Autodesk Inventor part; units mm, degrees
(part 2 of 4)
sketch "Sketch11" plane through (0, 0, -1) normal (0, 0, -1) x (-1, 0, 0)
  line L0 (5.295, -1.6238) -> (2.667, -1.6238) construction
  line L1 (2.667, -1.6238) -> (2.667, -0.5776) construction
  line L2 (2.667, -0.5776) -> (5.295, -0.5776) construction
  line L3 (5.295, -0.5776) -> (5.295, -1.6238) construction
  spline S0 degree 2 poles (4.8882, -1.2818) (4.8882, -1.2425) (4.915, -1.176) (4.9413, -1.1521) knots 0 0 0 1 2 2 2
  spline S1 degree 2 poles (4.9413, -1.1521) (4.9676, -1.1282) (5.0398, -1.1019) (5.0924, -1.1019) knots 0 0 0 1 2 2 2
  spline S2 degree 2 poles (5.0924, -1.1019) (5.1484, -1.1023) (5.2286, -1.1205) (5.2549, -1.1323) knots 0 0 0 1 2 2 2
  line L4 (5.2549, -1.1323) -> (5.2549, -1.2413)
  line L5 (5.2549, -1.2413) -> (5.2436, -1.2413)
  spline S3 degree 2 poles (5.2436, -1.2413) (5.2338, -1.236) (5.2103, -1.2222) (5.1913, -1.2149) knots 0 0 0 1 2 2 2
  spline S4 degree 2 poles (5.1913, -1.2149) (5.1735, -1.208) (5.1366, -1.1987) (5.1143, -1.1987) knots 0 0 0 1 2 2 2
  spline S5 degree 2 poles (5.1143, -1.1987) (5.0949, -1.1987) (5.0495, -1.2084) (5.0357, -1.2214) knots 0 0 0 1 2 2 2
  spline S6 degree 2 poles (5.0357, -1.2214) (5.0256, -1.2315) (5.0142, -1.2563) (5.0142, -1.2769) knots 0 0 0 1 2 2 2
  spline S7 degree 2 poles (5.0142, -1.2769) (5.0142, -1.2948) (5.0288, -1.3199) (5.0406, -1.3276) knots 0 0 0 1 2 2 2
  spline S8 degree 2 poles (5.0406, -1.3276) (5.0576, -1.3389) (5.1062, -1.3454) (5.1236, -1.3454) knots 0 0 0 1 2 2 2
  spline S9 degree 2 poles (5.1236, -1.3454) (5.1512, -1.3454) (5.2035, -1.3365) (5.2225, -1.3316) knots 0 0 0 1 2 2 2
  line L6 (5.2225, -1.3316) -> (5.2334, -1.3316)
  line L7 (5.2334, -1.3316) -> (5.2334, -1.6124)
  line L8 (5.2334, -1.6124) -> (4.902, -1.6124)
  line L9 (4.902, -1.6124) -> (4.902, -1.518)
  line L10 (4.902, -1.518) -> (5.1147, -1.518)
  line L11 (5.1147, -1.518) -> (5.1147, -1.4349)
  spline S10 degree 2 poles (5.1147, -1.4349) (5.1046, -1.4358) (5.0766, -1.4366) (5.0689, -1.4366) knots 0 0 0 1 2 2 2
  spline S11 degree 2 poles (5.0689, -1.4366) (5.0329, -1.4366) (4.9721, -1.422) (4.9482, -1.407) knots 0 0 0 1 2 2 2
  spline S12 degree 2 poles (4.9482, -1.407) (4.9198, -1.3883) (4.8882, -1.3264) (4.8882, -1.2818) knots 0 0 0 1 2 2 2
  spline S13 degree 2 poles (4.4401, -1.2514) (4.4401, -1.2194) (4.4668, -1.1639) (4.4924, -1.1436) knots 0 0 0 1 2 2 2
  spline S14 degree 2 poles (4.4924, -1.1436) (4.5179, -1.1234) (4.5912, -1.1007) (4.6386, -1.1007) knots 0 0 0 1 2 2 2
  spline S15 degree 2 poles (4.6386, -1.1007) (4.6893, -1.1007) (4.765, -1.1238) (4.7894, -1.1436) knots 0 0 0 1 2 2 2
  spline S16 degree 2 poles (4.7894, -1.1436) (4.8133, -1.1635) (4.836, -1.2174) (4.836, -1.2473) knots 0 0 0 1 2 2 2
  spline S17 degree 2 poles (4.836, -1.2473) (4.836, -1.2903) (4.7885, -1.3474) (4.7436, -1.3665) knots 0 0 0 1 2 2 2
  line L12 (4.7436, -1.3665) -> (4.7436, -1.3685)
  spline S18 degree 2 poles (4.7436, -1.3685) (4.7877, -1.39) (4.8226, -1.4512) (4.8226, -1.4888) knots 0 0 0 1 2 2 2
  spline S19 degree 2 poles (4.8226, -1.4888) (4.8226, -1.5164) (4.7983, -1.5646) (4.7744, -1.5836) knots 0 0 0 1 2 2 2
  spline S20 degree 2 poles (4.7744, -1.5836) (4.7513, -1.6019) (4.6812, -1.6238) (4.6374, -1.6238) knots 0 0 0 1 2 2 2
  spline S21 degree 2 poles (4.6374, -1.6238) (4.5912, -1.6238) (4.5223, -1.6039) (4.5001, -1.5877) knots 0 0 0 1 2 2 2
  spline S22 degree 2 poles (4.5001, -1.5877) (4.4774, -1.5715) (4.4531, -1.5245) (4.4531, -1.4973) knots 0 0 0 1 2 2 2
  spline S23 degree 2 poles (4.4531, -1.4973) (4.4531, -1.4617) (4.4944, -1.4046) (4.5369, -1.3847) knots 0 0 0 1 2 2 2
  line L13 (4.5369, -1.3847) -> (4.5369, -1.3831)
  spline S24 degree 2 poles (4.5369, -1.3831) (4.4871, -1.3628) (4.4401, -1.2972) (4.4401, -1.2514) knots 0 0 0 1 2 2 2
  spline S25 degree 2 poles (4.5641, -1.2461) (4.5641, -1.2708) (4.5851, -1.2968) (4.6192, -1.3134) knots 0 0 0 1 2 2 2
  spline S26 degree 2 poles (4.6192, -1.3134) (4.6289, -1.3178) (4.6658, -1.332) (4.68, -1.3381) knots 0 0 0 1 2 2 2
  spline S27 degree 2 poles (4.68, -1.3381) (4.6929, -1.3251) (4.7136, -1.2862) (4.7136, -1.2631) knots 0 0 0 1 2 2 2
  spline S28 degree 2 poles (4.7136, -1.2631) (4.7136, -1.2283) (4.669, -1.1866) (4.633, -1.1866) knots 0 0 0 1 2 2 2
  spline S29 degree 2 poles (4.633, -1.1866) (4.6228, -1.1866) (4.5977, -1.193) (4.588, -1.1995) knots 0 0 0 1 2 2 2
  spline S30 degree 2 poles (4.588, -1.1995) (4.577, -1.2072) (4.5641, -1.2283) (4.5641, -1.2461) knots 0 0 0 1 2 2 2
  spline S31 degree 2 poles (4.575, -1.4828) (4.575, -1.5083) (4.6086, -1.5387) (4.6374, -1.5387) knots 0 0 0 1 2 2 2
  spline S32 degree 2 poles (4.6374, -1.5387) (4.665, -1.5387) (4.6986, -1.5111) (4.6986, -1.4909) knots 0 0 0 1 2 2 2
  spline S33 degree 2 poles (4.6986, -1.4909) (4.6986, -1.471) (4.6783, -1.4463) (4.6569, -1.4362) knots 0 0 0 1 2 2 2
  spline S34 degree 2 poles (4.6569, -1.4362) (4.6475, -1.4313) (4.6216, -1.4212) (4.6001, -1.4131) knots 0 0 0 1 2 2 2
  spline S35 degree 2 poles (4.6001, -1.4131) (4.5872, -1.4301) (4.575, -1.4621) (4.575, -1.4828) knots 0 0 0 1 2 2 2
  line L14 (3.9948, -1.2291) -> (4.0625, -1.2291)
  line L15 (4.0625, -1.2291) -> (4.0625, -1.1112)
  line L16 (4.0625, -1.1112) -> (4.1836, -1.1112)
  line L17 (4.1836, -1.1112) -> (4.1836, -1.2291)
  line L18 (4.1836, -1.2291) -> (4.404, -1.2291)
  line L19 (4.404, -1.2291) -> (4.404, -1.3223)
  line L20 (4.404, -1.3223) -> (4.1877, -1.6124)
  line L21 (4.1877, -1.6124) -> (4.0625, -1.6124)
  line L22 (4.0625, -1.6124) -> (4.0625, -1.3191)
  line L23 (4.0625, -1.3191) -> (3.9948, -1.3191)
  line L24 (3.9948, -1.3191) -> (3.9948, -1.2291)
  line L25 (4.1836, -1.3191) -> (4.1836, -1.4892)
  line L26 (4.1836, -1.4892) -> (4.3104, -1.3191)
  line L27 (4.3104, -1.3191) -> (4.1836, -1.3191)
  point P0 (0, 0)
  constraints: 2 other
extrude "Extrusion11" add sketch "Sketch11" along normal blind 0.02 bodies 8
sketch "Sketch12" plane through (0, 0, 0) normal (0, 0, -1) x (-1, 0, 0)
  line L0 (3.7, 4.96) -> (5.6, 4.96)
  line L1 (5.6, 4.96) -> (5.6, 5.76)
  line L2 (5.6, 5.76) -> (3.7, 5.76)
  line L3 (3.7, 5.76) -> (3.7, 4.96)
  line L4 (3.6421, 4.9021) -> (3.6421, 5.8179)
  line L5 (5.6579, 5.8179) -> (5.6579, 4.9021)
  line L6 (5.7362, 4.8238) -> (5.7362, 5.8962)
  line L7 (3.5638, 5.8962) -> (3.5638, 4.8238)
  line L8 (4.75, 4.8238) -> (4.75, 4.9021)
  line L9 (4.55, 4.8238) -> (4.55, 4.9021)
  line L10 (4.75, 5.8179) -> (4.75, 5.8962)
  line L11 (4.55, 5.8179) -> (4.55, 5.8962)
  line L12 (3.6421, 5.8179) -> (4.55, 5.8179)
  line L13 (4.75, 5.8179) -> (5.6579, 5.8179)
  line L14 (5.7362, 5.8962) -> (4.75, 5.8962)
  line L15 (4.55, 5.8962) -> (3.5638, 5.8962)
  line L16 (5.6579, 4.9021) -> (4.75, 4.9021)
  line L17 (4.55, 4.9021) -> (3.6421, 4.9021)
  line L18 (3.5638, 4.8238) -> (4.55, 4.8238)
  line L19 (4.75, 4.8238) -> (5.7362, 4.8238)
  line L20 (3.6421, 3.5421) -> (3.6421, 4.4579)
  line L21 (5.6579, 4.4579) -> (5.6579, 3.5421)
  line L22 (5.7362, 3.4638) -> (5.7362, 4.5362)
  line L23 (3.5638, 4.5362) -> (3.5638, 3.4638)
  line L24 (4.75, 3.4638) -> (4.75, 3.5421)
  line L25 (4.55, 3.4638) -> (4.55, 3.5421)
  line L26 (4.75, 4.4579) -> (4.75, 4.5362)
  line L27 (4.55, 4.4579) -> (4.55, 4.5362)
  line L28 (3.6421, 4.4579) -> (4.55, 4.4579)
  line L29 (4.75, 4.4579) -> (5.6579, 4.4579)
  line L30 (5.7362, 4.5362) -> (4.75, 4.5362)
  line L31 (4.55, 4.5362) -> (3.5638, 4.5362)
  line L32 (5.6579, 3.5421) -> (4.75, 3.5421)
  line L33 (4.55, 3.5421) -> (3.6421, 3.5421)
  line L34 (3.5638, 3.4638) -> (4.55, 3.4638)
  line L35 (4.75, 3.4638) -> (5.7362, 3.4638)
  line L36 (3.6421, 2.2021) -> (3.6421, 3.1179)
  line L37 (5.6579, 3.1179) -> (5.6579, 2.2021)
  line L38 (5.7362, 2.1238) -> (5.7362, 3.1962)
  line L39 (3.5638, 3.1962) -> (3.5638, 2.1238)
  line L40 (4.75, 2.1238) -> (4.75, 2.2021)
  line L41 (4.55, 2.1238) -> (4.55, 2.2021)
  line L42 (4.75, 3.1179) -> (4.75, 3.1962)
  line L43 (4.55, 3.1179) -> (4.55, 3.1962)
  line L44 (3.6421, 3.1179) -> (4.55, 3.1179)
  line L45 (4.75, 3.1179) -> (5.6579, 3.1179)
  line L46 (5.7362, 3.1962) -> (4.75, 3.1962)
  line L47 (4.55, 3.1962) -> (3.5638, 3.1962)
  line L48 (5.6579, 2.2021) -> (4.75, 2.2021)
  line L49 (4.55, 2.2021) -> (3.6421, 2.2021)
  line L50 (3.5638, 2.1238) -> (4.55, 2.1238)
  line L51 (4.75, 2.1238) -> (5.7362, 2.1238)
  line L52 (3.6421, 0.8621) -> (3.6421, 1.7779)
  line L53 (5.6579, 1.7779) -> (5.6579, 0.8621)
  line L54 (5.7362, 0.7838) -> (5.7362, 1.8562)
  line L55 (3.5638, 1.8562) -> (3.5638, 0.7838)
  line L56 (4.75, 0.7838) -> (4.75, 0.8621)
  line L57 (4.55, 0.7838) -> (4.55, 0.8621)
  line L58 (4.75, 1.7779) -> (4.75, 1.8562)
  line L59 (4.55, 1.7779) -> (4.55, 1.8562)
  line L60 (3.6421, 1.7779) -> (4.55, 1.7779)
  line L61 (4.75, 1.7779) -> (5.6579, 1.7779)
  line L62 (5.7362, 1.8562) -> (4.75, 1.8562)
  line L63 (4.55, 1.8562) -> (3.5638, 1.8562)
  line L64 (5.6579, 0.8621) -> (4.75, 0.8621)
  line L65 (4.55, 0.8621) -> (3.6421, 0.8621)
  line L66 (3.5638, 0.7838) -> (4.55, 0.7838)
  line L67 (4.75, 0.7838) -> (5.7362, 0.7838)
  line L68 (3.6421, -0.4779) -> (3.6421, 0.4379)
  line L69 (5.6579, 0.4379) -> (5.6579, -0.4779)
  line L70 (5.7362, -0.5562) -> (5.7362, 0.5162)
  line L71 (3.5638, 0.5162) -> (3.5638, -0.5562)
  line L72 (4.75, -0.5562) -> (4.75, -0.4779)
  line L73 (4.55, -0.5562) -> (4.55, -0.4779)
  line L74 (4.75, 0.4379) -> (4.75, 0.5162)
  line L75 (4.55, 0.4379) -> (4.55, 0.5162)
  line L76 (3.6421, 0.4379) -> (4.55, 0.4379)
  line L77 (4.75, 0.4379) -> (5.6579, 0.4379)
  line L78 (5.7362, 0.5162) -> (4.75, 0.5162)
  line L79 (4.55, 0.5162) -> (3.5638, 0.5162)
  line L80 (5.6579, -0.4779) -> (4.75, -0.4779)
  line L81 (4.55, -0.4779) -> (3.6421, -0.4779)
  line L82 (3.5638, -0.5562) -> (4.55, -0.5562)
  line L83 (4.75, -0.5562) -> (5.7362, -0.5562)
  line L84 (3.6421, -1.8179) -> (3.6421, -0.9021)
  line L85 (5.6579, -0.9021) -> (5.6579, -1.8179)
  line L86 (5.7362, -1.8962) -> (5.7362, -0.8238)
  line L87 (3.5638, -0.8238) -> (3.5638, -1.8962)
  line L88 (4.75, -1.8962) -> (4.75, -1.8179)
  line L89 (4.55, -1.8962) -> (4.55, -1.8179)
  line L90 (4.75, -0.9021) -> (4.75, -0.8238)
  line L91 (4.55, -0.9021) -> (4.55, -0.8238)
  line L92 (3.6421, -0.9021) -> (4.55, -0.9021)
  line L93 (4.75, -0.9021) -> (5.6579, -0.9021)
  line L94 (5.7362, -0.8238) -> (4.75, -0.8238)
  line L95 (4.55, -0.8238) -> (3.5638, -0.8238)
  line L96 (5.6579, -1.8179) -> (4.75, -1.8179)
  line L97 (4.55, -1.8179) -> (3.6421, -1.8179)
  line L98 (3.5638, -1.8962) -> (4.55, -1.8962)
  line L99 (4.75, -1.8962) -> (5.7362, -1.8962)
  line L100 (3.6421, -3.1579) -> (3.6421, -2.2421)
  line L101 (5.6579, -2.2421) -> (5.6579, -3.1579)
  line L102 (5.7362, -3.2362) -> (5.7362, -2.1638)
  line L103 (3.5638, -2.1638) -> (3.5638, -3.2362)
  line L104 (4.75, -3.2362) -> (4.75, -3.1579)
  line L105 (4.55, -3.2362) -> (4.55, -3.1579)
  line L106 (4.75, -2.2421) -> (4.75, -2.1638)
  line L107 (4.55, -2.2421) -> (4.55, -2.1638)
  line L108 (3.6421, -2.2421) -> (4.55, -2.2421)
  line L109 (4.75, -2.2421) -> (5.6579, -2.2421)
  line L110 (5.7362, -2.1638) -> (4.75, -2.1638)
  line L111 (4.55, -2.1638) -> (3.5638, -2.1638)
  line L112 (5.6579, -3.1579) -> (4.75, -3.1579)
  line L113 (4.55, -3.1579) -> (3.6421, -3.1579)
  line L114 (3.5638, -3.2362) -> (4.55, -3.2362)
  line L115 (4.75, -3.2362) -> (5.7362, -3.2362)
  line L116 (3.6421, -4.4979) -> (3.6421, -3.5821)
  line L117 (5.6579, -3.5821) -> (5.6579, -4.4979)
  line L118 (5.7362, -4.5762) -> (5.7362, -3.5038)
  line L119 (3.5638, -3.5038) -> (3.5638, -4.5762)
  line L120 (4.75, -4.5762) -> (4.75, -4.4979)
  line L121 (4.55, -4.5762) -> (4.55, -4.4979)
  line L122 (4.75, -3.5821) -> (4.75, -3.5038)
  line L123 (4.55, -3.5821) -> (4.55, -3.5038)
  line L124 (3.6421, -3.5821) -> (4.55, -3.5821)
  line L125 (4.75, -3.5821) -> (5.6579, -3.5821)
  line L126 (5.7362, -3.5038) -> (4.75, -3.5038)
  line L127 (4.55, -3.5038) -> (3.5638, -3.5038)
  line L128 (5.6579, -4.4979) -> (4.75, -4.4979)
  line L129 (4.55, -4.4979) -> (3.6421, -4.4979)
  line L130 (3.5638, -4.5762) -> (4.55, -4.5762)
  line L131 (4.75, -4.5762) -> (5.7362, -4.5762)
  line L132 (3.6421, -5.8379) -> (3.6421, -4.9221)
  line L133 (5.6579, -4.9221) -> (5.6579, -5.8379)
  line L134 (5.7362, -5.9162) -> (5.7362, -4.8438)
  line L135 (3.5638, -4.8438) -> (3.5638, -5.9162)
  line L136 (4.75, -5.9162) -> (4.75, -5.8379)
  line L137 (4.55, -5.9162) -> (4.55, -5.8379)
  line L138 (4.75, -4.9221) -> (4.75, -4.8438)
  line L139 (4.55, -4.9221) -> (4.55, -4.8438)
  line L140 (3.6421, -4.9221) -> (4.55, -4.9221)
  line L141 (4.75, -4.9221) -> (5.6579, -4.9221)
  line L142 (5.7362, -4.8438) -> (4.75, -4.8438)
  line L143 (4.55, -4.8438) -> (3.5638, -4.8438)
  line L144 (5.6579, -5.8379) -> (4.75, -5.8379)
  line L145 (4.55, -5.8379) -> (3.6421, -5.8379)
  line L146 (3.5638, -5.9162) -> (4.55, -5.9162)
  line L147 (4.75, -5.9162) -> (5.7362, -5.9162)
  point P0 (0, 0)
  point P1 (5.6, 4.4)
  point P2 (5.6, 3.06)
  point P3 (5.6, 1.72)
  point P4 (5.6, 0.38)
  point P5 (5.6, -0.96)
  point P6 (5.6, -2.3)
  point P7 (5.6, -3.64)
  point P8 (5.6, -4.98)
  constraints: 288 end point
extrude "Extrusion12" add sketch "Sketch12" along normal blind 0.02 separate body contours L17 L9 L18 L7 L15 L11 L12 L4 | L13 L10 L14 L6 L19 L8 L16 L5 | L33 L25 L34 L23 L31 L27 L28 L20 | L29 L26 L30 L22 L35 L24 L32 L21 | L49 L41 L50 L39 L47 L43 L44 L36 | L45 L42 L46 L38 L51 L40 L48 L37 | L65 L57 L66 L55 L63 L59 L60 L52 | L61 L58 L62 L54 L67 L56 L64 L53 | L81 L73 L82 L71 L79 L75 L76 L68 | L77 L74 L78 L70 L83 L72 L80 L69 | L97 L89 L98 L87 L95 L91 L92 L84 | L93 L90 L94 L86 L99 L88 L96 L85 | L113 L105 L114 L103 L111 L107 L108 L100 | L109 L106 L110 L102 L115 L104 L112 L101 | L129 L121 L130 L119 L127 L123 L124 L116 | L125 L122 L126 L118 L131 L120 L128 L117 | L145 L137 L146 L135 L143 L139 L140 L132 | L141 L138 L142 L134 L147 L136 L144 L133
sketch "Sketch13" plane through (0, 0, 0) normal (0, 0, -1) x (-1, 0, 0)
  line L0 (5.9785, 5.8245) -> (7.8529, 5.8245) construction
  line L1 (7.8529, 5.8245) -> (7.8529, -6.7413) construction
  line L2 (7.8529, -6.7413) -> (5.9785, -6.7413) construction
  line L3 (5.9785, -6.7413) -> (5.9785, 5.8245) construction
  spline S0 degree 2 poles (6.5134, 4.784) (6.2881, 4.784) (6.0239, 5.0563) (6.0239, 5.3027) knots 0 0 0 1 2 2 2
  spline S1 degree 2 poles (6.0239, 5.3027) (6.0239, 5.5401) (6.2889, 5.8229) (6.5142, 5.8229) knots 0 0 0 1 2 2 2
  spline S2 degree 2 poles (6.5142, 5.8229) (6.5734, 5.8229) (6.669, 5.8091) (6.7127, 5.7978) knots 0 0 0 1 2 2 2
  spline S3 degree 2 poles (6.7127, 5.7978) (6.7468, 5.7873) (6.827, 5.7524) (6.8521, 5.7394) knots 0 0 0 1 2 2 2
  line L4 (6.8521, 5.7394) -> (6.8521, 5.5012)
  line L5 (6.8521, 5.5012) -> (6.827, 5.5012)
  spline S4 degree 2 poles (6.827, 5.5012) (6.8084, 5.5174) (6.7533, 5.5628) (6.7184, 5.5839) knots 0 0 0 1 2 2 2
  spline S5 degree 2 poles (6.7184, 5.5839) (6.6836, 5.6057) (6.6001, 5.6357) (6.5539, 5.6357) knots 0 0 0 1 2 2 2
  spline S6 degree 2 poles (6.5539, 5.6357) (6.4996, 5.6357) (6.4097, 5.6017) (6.3683, 5.5587) knots 0 0 0 1 2 2 2
  spline S7 degree 2 poles (6.3683, 5.5587) (6.3311, 5.5206) (6.2832, 5.3902) (6.2832, 5.3018) knots 0 0 0 1 2 2 2
  spline S8 degree 2 poles (6.2832, 5.3018) (6.2832, 5.2086) (6.3327, 5.0814) (6.3732, 5.0425) knots 0 0 0 1 2 2 2
  spline S9 degree 2 poles (6.3732, 5.0425) (6.4121, 5.0044) (6.5077, 4.9712) (6.5555, 4.9712) knots 0 0 0 1 2 2 2
  spline S10 degree 2 poles (6.5555, 4.9712) (6.605, 4.9712) (6.6949, 5.0044) (6.7257, 5.0247) knots 0 0 0 1 2 2 2
  spline S11 degree 2 poles (6.7257, 5.0247) (6.7597, 5.045) (6.8108, 5.0879) (6.8294, 5.1049) knots 0 0 0 1 2 2 2
  line L6 (6.8294, 5.1049) -> (6.8521, 5.1049)
  line L7 (6.8521, 5.1049) -> (6.8521, 4.8699)
  spline S12 degree 2 poles (6.8521, 4.8699) (6.8246, 4.8569) (6.7524, 4.8245) (6.7136, 4.8132) knots 0 0 0 1 2 2 2
  spline S13 degree 2 poles (6.7136, 4.8132) (6.6665, 4.7986) (6.5847, 4.784) (6.5134, 4.784) knots 0 0 0 1 2 2 2
  spline S14 degree 2 poles (7.7079, 5.1065) (7.7079, 5.0328) (7.6536, 4.9121) (7.6009, 4.8699) knots 0 0 0 1 2 2 2
  spline S15 degree 2 poles (7.6009, 4.8699) (7.5482, 4.8278) (7.4048, 4.7824) (7.3019, 4.7824) knots 0 0 0 1 2 2 2
  spline S16 degree 2 poles (7.3019, 4.7824) (7.1852, 4.7824) (7.0183, 4.8213) (6.9656, 4.8456) knots 0 0 0 1 2 2 2
  line L8 (6.9656, 4.8456) -> (6.9656, 5.0628)
  line L9 (6.9656, 5.0628) -> (6.9899, 5.0628)
  spline S17 degree 2 poles (6.9899, 5.0628) (7.045, 5.0279) (7.1933, 4.9761) (7.2549, 4.9761) knots 0 0 0 1 2 2 2
  spline S18 degree 2 poles (7.2549, 4.9761) (7.2913, 4.9761) (7.3764, 4.989) (7.4056, 5.0101) knots 0 0 0 1 2 2 2
  spline S19 degree 2 poles (7.4056, 5.0101) (7.4283, 5.0271) (7.4559, 5.0766) (7.4559, 5.1211) knots 0 0 0 1 2 2 2
  spline S20 degree 2 poles (7.4559, 5.1211) (7.4559, 5.1657) (7.417, 5.2135) (7.3845, 5.2249) knots 0 0 0 1 2 2 2
  spline S21 degree 2 poles (7.3845, 5.2249) (7.3521, 5.2362) (7.2622, 5.2386) (7.2273, 5.2386) knots 0 0 0 1 2 2 2
  line L10 (7.2273, 5.2386) -> (7.1844, 5.2386)
  line L11 (7.1844, 5.2386) -> (7.1844, 5.4145)
  line L12 (7.1844, 5.4145) -> (7.2241, 5.4145)
  spline S22 degree 2 poles (7.2241, 5.4145) (7.2695, 5.4145) (7.3465, 5.4226) (7.3732, 5.4347) knots 0 0 0 1 2 2 2
  spline S23 degree 2 poles (7.3732, 5.4347) (7.3999, 5.4477) (7.4299, 5.4931) (7.4299, 5.532) knots 0 0 0 1 2 2 2
  spline S24 degree 2 poles (7.4299, 5.532) (7.4299, 5.5628) (7.4016, 5.6009) (7.3813, 5.6114) knots 0 0 0 1 2 2 2
  spline S25 degree 2 poles (7.3813, 5.6114) (7.357, 5.6236) (7.2922, 5.6317) (7.2695, 5.6317) knots 0 0 0 1 2 2 2
  spline S26 degree 2 poles (7.2695, 5.6317) (7.233, 5.6317) (7.156, 5.6146) (7.1204, 5.6009) knots 0 0 0 1 2 2 2
  spline S27 degree 2 poles (7.1204, 5.6009) (7.092, 5.5903) (7.0304, 5.5563) (7.0158, 5.5474) knots 0 0 0 1 2 2 2
  line L13 (7.0158, 5.5474) -> (6.9948, 5.5474)
  line L14 (6.9948, 5.5474) -> (6.9948, 5.7613)
  spline S28 degree 2 poles (6.9948, 5.7613) (7.0466, 5.7832) (7.2217, 5.8245) (7.3132, 5.8245) knots 0 0 0 1 2 2 2
  spline S29 degree 2 poles (7.3132, 5.8245) (7.4024, 5.8245) (7.5336, 5.7937) (7.5798, 5.7638) knots 0 0 0 1 2 2 2
  spline S30 degree 2 poles (7.5798, 5.7638) (7.6309, 5.7321) (7.6819, 5.6349) (7.6819, 5.5741) knots 0 0 0 1 2 2 2
  spline S31 degree 2 poles (7.6819, 5.5741) (7.6819, 5.4882) (7.5831, 5.3602) (7.502, 5.3416) knots 0 0 0 1 2 2 2
  line L15 (7.502, 5.3416) -> (7.502, 5.3318)
  spline S32 degree 2 poles (7.502, 5.3318) (7.5377, 5.327) (7.6058, 5.301) (7.6382, 5.2719) knots 0 0 0 1 2 2 2
  spline S33 degree 2 poles (7.6382, 5.2719) (7.6682, 5.2459) (7.7079, 5.1633) (7.7079, 5.1065) knots 0 0 0 1 2 2 2
  spline S34 degree 2 poles (6.5134, 3.284) (6.2881, 3.284) (6.0239, 3.5563) (6.0239, 3.8027) knots 0 0 0 1 2 2 2
  spline S35 degree 2 poles (6.0239, 3.8027) (6.0239, 4.0401) (6.2889, 4.3229) (6.5142, 4.3229) knots 0 0 0 1 2 2 2
  spline S36 degree 2 poles (6.5142, 4.3229) (6.5734, 4.3229) (6.669, 4.3091) (6.7127, 4.2978) knots 0 0 0 1 2 2 2
  spline S37 degree 2 poles (6.7127, 4.2978) (6.7468, 4.2873) (6.827, 4.2524) (6.8521, 4.2394) knots 0 0 0 1 2 2 2
  line L16 (6.8521, 4.2394) -> (6.8521, 4.0012)
  line L17 (6.8521, 4.0012) -> (6.827, 4.0012)
  spline S38 degree 2 poles (6.827, 4.0012) (6.8084, 4.0174) (6.7533, 4.0628) (6.7184, 4.0839) knots 0 0 0 1 2 2 2
  spline S39 degree 2 poles (6.7184, 4.0839) (6.6836, 4.1057) (6.6001, 4.1357) (6.5539, 4.1357) knots 0 0 0 1 2 2 2
  spline S40 degree 2 poles (6.5539, 4.1357) (6.4996, 4.1357) (6.4097, 4.1017) (6.3683, 4.0587) knots 0 0 0 1 2 2 2
  spline S41 degree 2 poles (6.3683, 4.0587) (6.3311, 4.0206) (6.2832, 3.8902) (6.2832, 3.8018) knots 0 0 0 1 2 2 2
  spline S42 degree 2 poles (6.2832, 3.8018) (6.2832, 3.7086) (6.3327, 3.5814) (6.3732, 3.5425) knots 0 0 0 1 2 2 2
  spline S43 degree 2 poles (6.3732, 3.5425) (6.4121, 3.5044) (6.5077, 3.4712) (6.5555, 3.4712) knots 0 0 0 1 2 2 2
  spline S44 degree 2 poles (6.5555, 3.4712) (6.605, 3.4712) (6.6949, 3.5044) (6.7257, 3.5247) knots 0 0 0 1 2 2 2
  spline S45 degree 2 poles (6.7257, 3.5247) (6.7597, 3.545) (6.8108, 3.5879) (6.8294, 3.6049) knots 0 0 0 1 2 2 2
  line L18 (6.8294, 3.6049) -> (6.8521, 3.6049)
  line L19 (6.8521, 3.6049) -> (6.8521, 3.3699)
  spline S46 degree 2 poles (6.8521, 3.3699) (6.8246, 3.3569) (6.7524, 3.3245) (6.7136, 3.3132) knots 0 0 0 1 2 2 2
  spline S47 degree 2 poles (6.7136, 3.3132) (6.6665, 3.2986) (6.5847, 3.284) (6.5134, 3.284) knots 0 0 0 1 2 2 2
  line L20 (7.7452, 3.5368) -> (7.6098, 3.5368)
  line L21 (7.6098, 3.5368) -> (7.6098, 3.301)
  line L22 (7.6098, 3.301) -> (7.3675, 3.301)
  line L23 (7.3675, 3.301) -> (7.3675, 3.5368)
  line L24 (7.3675, 3.5368) -> (6.9267, 3.5368)
  line L25 (6.9267, 3.5368) -> (6.9267, 3.7232)
  line L26 (6.9267, 3.7232) -> (7.3594, 4.3035)
  line L27 (7.3594, 4.3035) -> (7.6098, 4.3035)
  line L28 (7.6098, 4.3035) -> (7.6098, 3.7168)
  line L29 (7.6098, 3.7168) -> (7.7452, 3.7168)
  line L30 (7.7452, 3.7168) -> (7.7452, 3.5368)
  line L31 (7.3675, 3.7168) -> (7.3675, 4.0571)
  line L32 (7.3675, 4.0571) -> (7.1139, 3.7168)
  line L33 (7.1139, 3.7168) -> (7.3675, 3.7168)
  spline S48 degree 2 poles (6.5134, 1.784) (6.2881, 1.784) (6.0239, 2.0563) (6.0239, 2.3027) knots 0 0 0 1 2 2 2
  spline S49 degree 2 poles (6.0239, 2.3027) (6.0239, 2.5401) (6.2889, 2.8229) (6.5142, 2.8229) knots 0 0 0 1 2 2 2
  spline S50 degree 2 poles (6.5142, 2.8229) (6.5734, 2.8229) (6.669, 2.8091) (6.7127, 2.7978) knots 0 0 0 1 2 2 2
  spline S51 degree 2 poles (6.7127, 2.7978) (6.7468, 2.7873) (6.827, 2.7524) (6.8521, 2.7394) knots 0 0 0 1 2 2 2
  line L34 (6.8521, 2.7394) -> (6.8521, 2.5012)
  line L35 (6.8521, 2.5012) -> (6.827, 2.5012)
  spline S52 degree 2 poles (6.827, 2.5012) (6.8084, 2.5174) (6.7533, 2.5628) (6.7184, 2.5839) knots 0 0 0 1 2 2 2
  spline S53 degree 2 poles (6.7184, 2.5839) (6.6836, 2.6057) (6.6001, 2.6357) (6.5539, 2.6357) knots 0 0 0 1 2 2 2
  spline S54 degree 2 poles (6.5539, 2.6357) (6.4996, 2.6357) (6.4097, 2.6017) (6.3683, 2.5587) knots 0 0 0 1 2 2 2
  spline S55 degree 2 poles (6.3683, 2.5587) (6.3311, 2.5206) (6.2832, 2.3902) (6.2832, 2.3018) knots 0 0 0 1 2 2 2
  spline S56 degree 2 poles (6.2832, 2.3018) (6.2832, 2.2086) (6.3327, 2.0814) (6.3732, 2.0425) knots 0 0 0 1 2 2 2
  spline S57 degree 2 poles (6.3732, 2.0425) (6.4121, 2.0044) (6.5077, 1.9712) (6.5555, 1.9712) knots 0 0 0 1 2 2 2
  spline S58 degree 2 poles (6.5555, 1.9712) (6.605, 1.9712) (6.6949, 2.0044) (6.7257, 2.0247) knots 0 0 0 1 2 2 2
  spline S59 degree 2 poles (6.7257, 2.0247) (6.7597, 2.045) (6.8108, 2.0879) (6.8294, 2.1049) knots 0 0 0 1 2 2 2
  line L36 (6.8294, 2.1049) -> (6.8521, 2.1049)
  line L37 (6.8521, 2.1049) -> (6.8521, 1.8699)
  spline S60 degree 2 poles (6.8521, 1.8699) (6.8246, 1.8569) (6.7524, 1.8245) (6.7136, 1.8132) knots 0 0 0 1 2 2 2
  spline S61 degree 2 poles (6.7136, 1.8132) (6.6665, 1.7986) (6.5847, 1.784) (6.5134, 1.784) knots 0 0 0 1 2 2 2
  line L38 (7.6884, 1.8035) -> (7.028, 1.8035)
  line L39 (7.028, 1.8035) -> (7.028, 1.9777)
  line L40 (7.028, 1.9777) -> (7.2387, 1.9777)
  line L41 (7.2387, 1.9777) -> (7.2387, 2.5069)
  line L42 (7.2387, 2.5069) -> (7.028, 2.5069)
  line L43 (7.028, 2.5069) -> (7.028, 2.6698)
  spline S62 degree 2 poles (7.028, 2.6698) (7.0742, 2.6698) (7.1657, 2.6819) (7.1933, 2.6949) knots 0 0 0 1 2 2 2
  spline S63 degree 2 poles (7.1933, 2.6949) (7.2249, 2.7111) (7.2606, 2.7654) (7.2638, 2.8059) knots 0 0 0 1 2 2 2
  line L44 (7.2638, 2.8059) -> (7.4826, 2.8059)
  line L45 (7.4826, 2.8059) -> (7.4826, 1.9777)
  line L46 (7.4826, 1.9777) -> (7.6884, 1.9777)
  line L47 (7.6884, 1.9777) -> (7.6884, 1.8035)
  spline S64 degree 2 poles (6.5134, 0.284) (6.2881, 0.284) (6.0239, 0.5563) (6.0239, 0.8027) knots 0 0 0 1 2 2 2
  spline S65 degree 2 poles (6.0239, 0.8027) (6.0239, 1.0401) (6.2889, 1.3229) (6.5142, 1.3229) knots 0 0 0 1 2 2 2
  spline S66 degree 2 poles (6.5142, 1.3229) (6.5734, 1.3229) (6.669, 1.3091) (6.7127, 1.2978) knots 0 0 0 1 2 2 2
  spline S67 degree 2 poles (6.7127, 1.2978) (6.7468, 1.2873) (6.827, 1.2524) (6.8521, 1.2394) knots 0 0 0 1 2 2 2
  line L48 (6.8521, 1.2394) -> (6.8521, 1.0012)
  line L49 (6.8521, 1.0012) -> (6.827, 1.0012)
  spline S68 degree 2 poles (6.827, 1.0012) (6.8084, 1.0174) (6.7533, 1.0628) (6.7184, 1.0839) knots 0 0 0 1 2 2 2
  spline S69 degree 2 poles (6.7184, 1.0839) (6.6836, 1.1057) (6.6001, 1.1357) (6.5539, 1.1357) knots 0 0 0 1 2 2 2
  spline S70 degree 2 poles (6.5539, 1.1357) (6.4996, 1.1357) (6.4097, 1.1017) (6.3683, 1.0587) knots 0 0 0 1 2 2 2
  spline S71 degree 2 poles (6.3683, 1.0587) (6.3311, 1.0206) (6.2832, 0.8902) (6.2832, 0.8018) knots 0 0 0 1 2 2 2
  spline S72 degree 2 poles (6.2832, 0.8018) (6.2832, 0.7086) (6.3327, 0.5814) (6.3732, 0.5425) knots 0 0 0 1 2 2 2
  spline S73 degree 2 poles (6.3732, 0.5425) (6.4121, 0.5044) (6.5077, 0.4712) (6.5555, 0.4712) knots 0 0 0 1 2 2 2
  spline S74 degree 2 poles (6.5555, 0.4712) (6.605, 0.4712) (6.6949, 0.5044) (6.7257, 0.5247) knots 0 0 0 1 2 2 2
  spline S75 degree 2 poles (6.7257, 0.5247) (6.7597, 0.545) (6.8108, 0.5879) (6.8294, 0.6049) knots 0 0 0 1 2 2 2
  line L50 (6.8294, 0.6049) -> (6.8521, 0.6049)
  line L51 (6.8521, 0.6049) -> (6.8521, 0.3699)
  spline S76 degree 2 poles (6.8521, 0.3699) (6.8246, 0.3569) (6.7524, 0.3245) (6.7136, 0.3132) knots 0 0 0 1 2 2 2
  spline S77 degree 2 poles (6.7136, 0.3132) (6.6665, 0.2986) (6.5847, 0.284) (6.5134, 0.284) knots 0 0 0 1 2 2 2
  line L52 (7.733, 0.3035) -> (6.998, 0.3035)
  line L53 (6.998, 0.3035) -> (6.998, 0.4663)
  spline S78 degree 2 poles (6.998, 0.4663) (7.0912, 0.5409) (7.2403, 0.6722) (7.2962, 0.7313) knots 0 0 0 1 2 2 2
  spline S79 degree 2 poles (7.2962, 0.7313) (7.37, 0.8083) (7.4356, 0.9258) (7.4356, 0.9874) knots 0 0 0 1 2 2 2
  spline S80 degree 2 poles (7.4356, 0.9874) (7.4356, 1.0571) (7.3521, 1.1317) (7.2776, 1.1317) knots 0 0 0 1 2 2 2
  spline S81 degree 2 poles (7.2776, 1.1317) (7.2395, 1.1317) (7.1714, 1.113) (7.1366, 1.0984) knots 0 0 0 1 2 2 2
  spline S82 degree 2 poles (7.1366, 1.0984) (7.1025, 1.083) (7.0539, 1.0506) (7.0418, 1.0425) knots 0 0 0 1 2 2 2
  line L54 (7.0418, 1.0425) -> (7.0223, 1.0425)
  line L55 (7.0223, 1.0425) -> (7.0223, 1.2605)
  spline S83 degree 2 poles (7.0223, 1.2605) (7.0644, 1.2808) (7.2443, 1.3229) (7.3278, 1.3229) knots 0 0 0 1 2 2 2
  spline S84 degree 2 poles (7.3278, 1.3229) (7.5061, 1.3229) (7.6892, 1.1641) (7.6892, 1.0206) knots 0 0 0 1 2 2 2
  spline S85 degree 2 poles (7.6892, 1.0206) (7.6892, 0.9323) (7.6058, 0.7621) (7.5093, 0.6649) knots 0 0 0 1 2 2 2
  spline S86 degree 2 poles (7.5093, 0.6649) (7.4486, 0.6049) (7.3343, 0.5117) (7.3092, 0.4923) knots 0 0 0 1 2 2 2
  line L56 (7.3092, 0.4923) -> (7.733, 0.4923)
  line L57 (7.733, 0.4923) -> (7.733, 0.3035)
  line L58 (7.0061, -1.1965) -> (6.7006, -1.1965)
  line L59 (6.7006, -1.1965) -> (6.4226, -0.8294)
  line L60 (6.4226, -0.8294) -> (6.3319, -0.8294)
  line L61 (6.3319, -0.8294) -> (6.3319, -1.1965)
  line L62 (6.3319, -1.1965) -> (6.0823, -1.1965)
  line L63 (6.0823, -1.1965) -> (6.0823, -0.1965)
  line L64 (6.0823, -0.1965) -> (6.4842, -0.1965)
  spline S87 degree 2 poles (6.4842, -0.1965) (6.5677, -0.1965) (6.6909, -0.2176) (6.7435, -0.25) knots 0 0 0 1 2 2 2
  spline S88 degree 2 poles (6.7435, -0.25) (6.797, -0.2841) (6.8602, -0.3902) (6.8602, -0.4713) knots 0 0 0 1 2 2 2
  spline S89 degree 2 poles (6.8602, -0.4713) (6.8602, -0.5855) (6.7565, -0.729) (6.6698, -0.7711) knots 0 0 0 1 2 2 2
  line L65 (6.6698, -0.7711) -> (7.0061, -1.1965)
  spline S90 degree 2 poles (6.6025, -0.5029) (6.6025, -0.4648) (6.5734, -0.4105) (6.5401, -0.3959) knots 0 0 0 1 2 2 2
  spline S91 degree 2 poles (6.5401, -0.3959) (6.5166, -0.3862) (6.4591, -0.3805) (6.4161, -0.3805) knots 0 0 0 1 2 2 2
  line L66 (6.4161, -0.3805) -> (6.3319, -0.3805)
  line L67 (6.3319, -0.3805) -> (6.3319, -0.6495)
  line L68 (6.3319, -0.6495) -> (6.404, -0.6495)
  spline S92 degree 2 poles (6.404, -0.6495) (6.4559, -0.6495) (6.5296, -0.6366) (6.5547, -0.6163) knots 0 0 0 1 2 2 2
  spline S93 degree 2 poles (6.5547, -0.6163) (6.579, -0.5969) (6.6025, -0.545) (6.6025, -0.5029) knots 0 0 0 1 2 2 2
  line L69 (7.7687, -1.1965) -> (7.1082, -1.1965)
  line L70 (7.1082, -1.1965) -> (7.1082, -1.0223)
  line L71 (7.1082, -1.0223) -> (7.3189, -1.0223)
  line L72 (7.3189, -1.0223) -> (7.3189, -0.4931)
  line L73 (7.3189, -0.4931) -> (7.1082, -0.4931)
  line L74 (7.1082, -0.4931) -> (7.1082, -0.3302)
  spline S94 degree 2 poles (7.1082, -0.3302) (7.1544, -0.3302) (7.246, -0.3181) (7.2735, -0.3051) knots 0 0 0 1 2 2 2
  spline S95 degree 2 poles (7.2735, -0.3051) (7.3051, -0.2889) (7.3408, -0.2346) (7.344, -0.1941) knots 0 0 0 1 2 2 2
  line L75 (7.344, -0.1941) -> (7.5628, -0.1941)
  line L76 (7.5628, -0.1941) -> (7.5628, -1.0223)
  line L77 (7.5628, -1.0223) -> (7.7687, -1.0223)
  line L78 (7.7687, -1.0223) -> (7.7687, -1.1965)
  spline S96 degree 2 poles (6.5134, -2.716) (6.2881, -2.716) (6.0239, -2.4437) (6.0239, -2.1973) knots 0 0 0 1 2 2 2
  spline S97 degree 2 poles (6.0239, -2.1973) (6.0239, -1.9599) (6.2889, -1.6771) (6.5142, -1.6771) knots 0 0 0 1 2 2 2
  spline S98 degree 2 poles (6.5142, -1.6771) (6.5734, -1.6771) (6.669, -1.6909) (6.7127, -1.7022) knots 0 0 0 1 2 2 2
  spline S99 degree 2 poles (6.7127, -1.7022) (6.7468, -1.7127) (6.827, -1.7476) (6.8521, -1.7606) knots 0 0 0 1 2 2 2
  line L79 (6.8521, -1.7606) -> (6.8521, -1.9988)
  line L80 (6.8521, -1.9988) -> (6.827, -1.9988)
  spline S100 degree 2 poles (6.827, -1.9988) (6.8084, -1.9826) (6.7533, -1.9372) (6.7184, -1.9161) knots 0 0 0 1 2 2 2
  spline S101 degree 2 poles (6.7184, -1.9161) (6.6836, -1.8943) (6.6001, -1.8643) (6.5539, -1.8643) knots 0 0 0 1 2 2 2
  spline S102 degree 2 poles (6.5539, -1.8643) (6.4996, -1.8643) (6.4097, -1.8983) (6.3683, -1.9413) knots 0 0 0 1 2 2 2
  spline S103 degree 2 poles (6.3683, -1.9413) (6.3311, -1.9794) (6.2832, -2.1098) (6.2832, -2.1982) knots 0 0 0 1 2 2 2
  spline S104 degree 2 poles (6.2832, -2.1982) (6.2832, -2.2914) (6.3327, -2.4186) (6.3732, -2.4575) knots 0 0 0 1 2 2 2
  spline S105 degree 2 poles (6.3732, -2.4575) (6.4121, -2.4956) (6.5077, -2.5288) (6.5555, -2.5288) knots 0 0 0 1 2 2 2
  spline S106 degree 2 poles (6.5555, -2.5288) (6.605, -2.5288) (6.6949, -2.4956) (6.7257, -2.4753) knots 0 0 0 1 2 2 2
  spline S107 degree 2 poles (6.7257, -2.4753) (6.7597, -2.455) (6.8108, -2.4121) (6.8294, -2.3951) knots 0 0 0 1 2 2 2
  line L81 (6.8294, -2.3951) -> (6.8521, -2.3951)
  line L82 (6.8521, -2.3951) -> (6.8521, -2.6301)
  spline S108 degree 2 poles (6.8521, -2.6301) (6.8246, -2.6431) (6.7524, -2.6755) (6.7136, -2.6868) knots 0 0 0 1 2 2 2
  spline S109 degree 2 poles (6.7136, -2.6868) (6.6665, -2.7014) (6.5847, -2.716) (6.5134, -2.716) knots 0 0 0 1 2 2 2
  spline S110 degree 2 poles (7.7103, -2.3578) (7.7103, -2.4364) (7.6568, -2.5693) (7.6042, -2.6171) knots 0 0 0 1 2 2 2
  spline S111 degree 2 poles (7.6042, -2.6171) (7.5515, -2.6649) (7.4072, -2.7176) (7.3019, -2.7176) knots 0 0 0 1 2 2 2
  spline S112 degree 2 poles (7.3019, -2.7176) (7.1901, -2.7168) (7.0296, -2.6803) (6.9769, -2.6568) knots 0 0 0 1 2 2 2
  line L83 (6.9769, -2.6568) -> (6.9769, -2.4388)
  line L84 (6.9769, -2.4388) -> (6.9996, -2.4388)
  spline S113 degree 2 poles (6.9996, -2.4388) (7.0191, -2.4494) (7.0661, -2.4769) (7.1042, -2.4915) knots 0 0 0 1 2 2 2
  spline S114 degree 2 poles (7.1042, -2.4915) (7.1398, -2.5053) (7.2136, -2.5239) (7.2581, -2.5239) knots 0 0 0 1 2 2 2
  spline S115 degree 2 poles (7.2581, -2.5239) (7.297, -2.5239) (7.3878, -2.5045) (7.4153, -2.4785) knots 0 0 0 1 2 2 2
  spline S116 degree 2 poles (7.4153, -2.4785) (7.4356, -2.4583) (7.4583, -2.4089) (7.4583, -2.3675) knots 0 0 0 1 2 2 2
  spline S117 degree 2 poles (7.4583, -2.3675) (7.4583, -2.3319) (7.4291, -2.2816) (7.4056, -2.2662) knots 0 0 0 1 2 2 2
  spline S118 degree 2 poles (7.4056, -2.2662) (7.3716, -2.2435) (7.2743, -2.2306) (7.2395, -2.2306) knots 0 0 0 1 2 2 2
  spline S119 degree 2 poles (7.2395, -2.2306) (7.1844, -2.2306) (7.0798, -2.2484) (7.0418, -2.2581) knots 0 0 0 1 2 2 2
  line L85 (7.0418, -2.2581) -> (7.0199, -2.2581)
  line L86 (7.0199, -2.2581) -> (7.0199, -1.6965)
  line L87 (7.0199, -1.6965) -> (7.6828, -1.6965)
  line L88 (7.6828, -1.6965) -> (7.6828, -1.8854)
  line L89 (7.6828, -1.8854) -> (7.2573, -1.8854)
  line L90 (7.2573, -1.8854) -> (7.2573, -2.0515)
  spline S120 degree 2 poles (7.2573, -2.0515) (7.2776, -2.0499) (7.3335, -2.0482) (7.3489, -2.0482) knots 0 0 0 1 2 2 2
  spline S121 degree 2 poles (7.3489, -2.0482) (7.421, -2.0482) (7.5426, -2.0774) (7.5904, -2.1074) knots 0 0 0 1 2 2 2
  spline S122 degree 2 poles (7.5904, -2.1074) (7.6471, -2.1447) (7.7103, -2.2687) (7.7103, -2.3578) knots 0 0 0 1 2 2 2
  spline S123 degree 2 poles (6.5134, -4.216) (6.2881, -4.216) (6.0239, -3.9437) (6.0239, -3.6973) knots 0 0 0 1 2 2 2
  spline S124 degree 2 poles (6.0239, -3.6973) (6.0239, -3.4599) (6.2889, -3.1771) (6.5142, -3.1771) knots 0 0 0 1 2 2 2
  spline S125 degree 2 poles (6.5142, -3.1771) (6.5734, -3.1771) (6.669, -3.1909) (6.7127, -3.2022) knots 0 0 0 1 2 2 2
  spline S126 degree 2 poles (6.7127, -3.2022) (6.7468, -3.2127) (6.827, -3.2476) (6.8521, -3.2606) knots 0 0 0 1 2 2 2
  line L91 (6.8521, -3.2606) -> (6.8521, -3.4988)
  line L92 (6.8521, -3.4988) -> (6.827, -3.4988)
  spline S127 degree 2 poles (6.827, -3.4988) (6.8084, -3.4826) (6.7533, -3.4372) (6.7184, -3.4161) knots 0 0 0 1 2 2 2
  spline S128 degree 2 poles (6.7184, -3.4161) (6.6836, -3.3943) (6.6001, -3.3643) (6.5539, -3.3643) knots 0 0 0 1 2 2 2
  spline S129 degree 2 poles (6.5539, -3.3643) (6.4996, -3.3643) (6.4097, -3.3983) (6.3683, -3.4413) knots 0 0 0 1 2 2 2
  spline S130 degree 2 poles (6.3683, -3.4413) (6.3311, -3.4794) (6.2832, -3.6098) (6.2832, -3.6982) knots 0 0 0 1 2 2 2
  spline S131 degree 2 poles (6.2832, -3.6982) (6.2832, -3.7914) (6.3327, -3.9186) (6.3732, -3.9575) knots 0 0 0 1 2 2 2
  spline S132 degree 2 poles (6.3732, -3.9575) (6.4121, -3.9956) (6.5077, -4.0288) (6.5555, -4.0288) knots 0 0 0 1 2 2 2
  spline S133 degree 2 poles (6.5555, -4.0288) (6.605, -4.0288) (6.6949, -3.9956) (6.7257, -3.9753) knots 0 0 0 1 2 2 2
  spline S134 degree 2 poles (6.7257, -3.9753) (6.7597, -3.955) (6.8108, -3.9121) (6.8294, -3.8951) knots 0 0 0 1 2 2 2
  line L93 (6.8294, -3.8951) -> (6.8521, -3.8951)
  line L94 (6.8521, -3.8951) -> (6.8521, -4.1301)
  spline S135 degree 2 poles (6.8521, -4.1301) (6.8246, -4.1431) (6.7524, -4.1755) (6.7136, -4.1868) knots 0 0 0 1 2 2 2
  spline S136 degree 2 poles (6.7136, -4.1868) (6.6665, -4.2014) (6.5847, -4.216) (6.5134, -4.216) knots 0 0 0 1 2 2 2
  spline S137 degree 2 poles (7.7306, -3.9186) (7.7306, -3.9826) (7.6771, -4.0936) (7.626, -4.1341) knots 0 0 0 1 2 2 2
  spline S138 degree 2 poles (7.626, -4.1341) (7.575, -4.1747) (7.4283, -4.22) (7.3335, -4.22) knots 0 0 0 1 2 2 2
  spline S139 degree 2 poles (7.3335, -4.22) (7.2322, -4.22) (7.0806, -4.1738) (7.032, -4.1341) knots 0 0 0 1 2 2 2
  spline S140 degree 2 poles (7.032, -4.1341) (6.9842, -4.0944) (6.9388, -3.9867) (6.9388, -3.9267) knots 0 0 0 1 2 2 2
  spline S141 degree 2 poles (6.9388, -3.9267) (6.9388, -3.8408) (7.0336, -3.7265) (7.1236, -3.6884) knots 0 0 0 1 2 2 2
  line L95 (7.1236, -3.6884) -> (7.1236, -3.6844)
  spline S142 degree 2 poles (7.1236, -3.6844) (7.0353, -3.6414) (6.9656, -3.5191) (6.9656, -3.4437) knots 0 0 0 1 2 2 2
  spline S143 degree 2 poles (6.9656, -3.4437) (6.9656, -3.3886) (7.0142, -3.2922) (7.062, -3.2541) knots 0 0 0 1 2 2 2
  spline S144 degree 2 poles (7.062, -3.2541) (7.1082, -3.2176) (7.2484, -3.1738) (7.3359, -3.1738) knots 0 0 0 1 2 2 2
  spline S145 degree 2 poles (7.3359, -3.1738) (7.4283, -3.1738) (7.5661, -3.2136) (7.6106, -3.246) knots 0 0 0 1 2 2 2
  spline S146 degree 2 poles (7.6106, -3.246) (7.656, -3.2784) (7.7046, -3.3724) (7.7046, -3.4267) knots 0 0 0 1 2 2 2
  spline S147 degree 2 poles (7.7046, -3.4267) (7.7046, -3.498) (7.622, -3.6123) (7.5369, -3.652) knots 0 0 0 1 2 2 2
  line L96 (7.5369, -3.652) -> (7.5369, -3.6552)
  spline S148 degree 2 poles (7.5369, -3.6552) (7.6366, -3.6957) (7.7306, -3.827) (7.7306, -3.9186) knots 0 0 0 1 2 2 2
  spline S149 degree 2 poles (7.4826, -3.9291) (7.4826, -3.8797) (7.4405, -3.8278) (7.3724, -3.7946) knots 0 0 0 1 2 2 2
  spline S150 degree 2 poles (7.3724, -3.7946) (7.3529, -3.7857) (7.2792, -3.7573) (7.2508, -3.7452) knots 0 0 0 1 2 2 2
  spline S151 degree 2 poles (7.2508, -3.7452) (7.2249, -3.7711) (7.1836, -3.8489) (7.1836, -3.8951) knots 0 0 0 1 2 2 2
  spline S152 degree 2 poles (7.1836, -3.8951) (7.1836, -3.9648) (7.2727, -4.0482) (7.3448, -4.0482) knots 0 0 0 1 2 2 2
  spline S153 degree 2 poles (7.3448, -4.0482) (7.3651, -4.0482) (7.4153, -4.0353) (7.4348, -4.0223) knots 0 0 0 1 2 2 2
  spline S154 degree 2 poles (7.4348, -4.0223) (7.4567, -4.0069) (7.4826, -3.9648) (7.4826, -3.9291) knots 0 0 0 1 2 2 2
  spline S155 degree 2 poles (7.4607, -3.4559) (7.4607, -3.4048) (7.3935, -3.344) (7.3359, -3.344) knots 0 0 0 1 2 2 2
  spline S156 degree 2 poles (7.3359, -3.344) (7.2808, -3.344) (7.2136, -3.3991) (7.2136, -3.4396) knots 0 0 0 1 2 2 2
  spline S157 degree 2 poles (7.2136, -3.4396) (7.2136, -3.4794) (7.2541, -3.5288) (7.297, -3.549) knots 0 0 0 1 2 2 2
  spline S158 degree 2 poles (7.297, -3.549) (7.3157, -3.5588) (7.3675, -3.579) (7.4105, -3.5952) knots 0 0 0 1 2 2 2
  spline S159 degree 2 poles (7.4105, -3.5952) (7.4364, -3.5612) (7.4607, -3.4972) (7.4607, -3.4559) knots 0 0 0 1 2 2 2
  spline S160 degree 2 poles (6.5134, -5.716) (6.2881, -5.716) (6.0239, -5.4437) (6.0239, -5.1973) knots 0 0 0 1 2 2 2
  spline S161 degree 2 poles (6.0239, -5.1973) (6.0239, -4.9599) (6.2889, -4.6771) (6.5142, -4.6771) knots 0 0 0 1 2 2 2
  spline S162 degree 2 poles (6.5142, -4.6771) (6.5734, -4.6771) (6.669, -4.6909) (6.7127, -4.7022) knots 0 0 0 1 2 2 2
  spline S163 degree 2 poles (6.7127, -4.7022) (6.7468, -4.7127) (6.827, -4.7476) (6.8521, -4.7606) knots 0 0 0 1 2 2 2
  line L97 (6.8521, -4.7606) -> (6.8521, -4.9988)
  line L98 (6.8521, -4.9988) -> (6.827, -4.9988)
  spline S164 degree 2 poles (6.827, -4.9988) (6.8084, -4.9826) (6.7533, -4.9372) (6.7184, -4.9161) knots 0 0 0 1 2 2 2
  spline S165 degree 2 poles (6.7184, -4.9161) (6.6836, -4.8943) (6.6001, -4.8643) (6.5539, -4.8643) knots 0 0 0 1 2 2 2
  spline S166 degree 2 poles (6.5539, -4.8643) (6.4996, -4.8643) (6.4097, -4.8983) (6.3683, -4.9413) knots 0 0 0 1 2 2 2
  spline S167 degree 2 poles (6.3683, -4.9413) (6.3311, -4.9794) (6.2832, -5.1098) (6.2832, -5.1982) knots 0 0 0 1 2 2 2
  spline S168 degree 2 poles (6.2832, -5.1982) (6.2832, -5.2914) (6.3327, -5.4186) (6.3732, -5.4575) knots 0 0 0 1 2 2 2
  spline S169 degree 2 poles (6.3732, -5.4575) (6.4121, -5.4956) (6.5077, -5.5288) (6.5555, -5.5288) knots 0 0 0 1 2 2 2
  spline S170 degree 2 poles (6.5555, -5.5288) (6.605, -5.5288) (6.6949, -5.4956) (6.7257, -5.4753) knots 0 0 0 1 2 2 2
  spline S171 degree 2 poles (6.7257, -5.4753) (6.7597, -5.455) (6.8108, -5.4121) (6.8294, -5.3951) knots 0 0 0 1 2 2 2
  line L99 (6.8294, -5.3951) -> (6.8521, -5.3951)
  line L100 (6.8521, -5.3951) -> (6.8521, -5.6301)
  spline S172 degree 2 poles (6.8521, -5.6301) (6.8246, -5.6431) (6.7524, -5.6755) (6.7136, -5.6868) knots 0 0 0 1 2 2 2
  spline S173 degree 2 poles (6.7136, -5.6868) (6.6665, -5.7014) (6.5847, -5.716) (6.5134, -5.716) knots 0 0 0 1 2 2 2
  line L101 (7.7111, -4.8951) -> (7.2841, -5.6965)
  line L102 (7.2841, -5.6965) -> (7.0053, -5.6965)
  line L103 (7.0053, -5.6965) -> (7.4518, -4.8854)
  line L104 (7.4518, -4.8854) -> (6.9753, -4.8854)
  line L105 (6.9753, -4.8854) -> (6.9753, -4.6965)
  line L106 (6.9753, -4.6965) -> (7.7111, -4.6965)
  line L107 (7.7111, -4.6965) -> (7.7111, -4.8951)
  point P0 (0, 0)
  constraints: 2 other
extrude "Extrusion13" add sketch "Sketch13" along normal blind 0.02 separate body